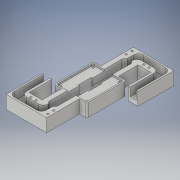
# Autodesk Inventor part: Enclosure_Bottom V6
Saved by Autodesk Inventor 2017 (Build 210142000, 142)
## iProperties
Created: 2017-11-29
Part Number: Enclosure_Bottom V6
Material: Generic
Document SubType Name: Modeling
Designer: Tripl_000
Density: 1 g/cm^3
Appearance: Default
Author: Tripl_000
Autodesk Inventor part; units mm, degrees
ref_plane "YZ Plane" through (0, 0, 0) normal (1, 0, 0) x (0, 1, 0)
ref_plane "XZ Plane" through (0, 0, 0) normal (0, 1, 0) x (-1, 0, 0)
ref_plane "XY Plane" through (0, 0, 0) normal (0, 0, 1) x (1, 0, 0)
sketch "Sketch1" plane through (0, 0, 0) normal (0, 1, 0) x (-1, 0, 0)
  line L0 (-25, 30) -> (25, 30)
  line L1 (25, 30) -> (25, -30)
  line L2 (25, -30) -> (-25, -30)
  line L3 (-25, -30) -> (-25, 30)
  line L4 (-25, 30) -> (25, -30) construction
  line L5 (25, 30) -> (-25, -30) construction
  point P0 (0, 0)
  dimension "d0" = 50
  dimension "d1" = 60
  constraints: 12 end point, 2 midpoint, 2 parallel, 1 horizontal, 1 perpendicular
  measures "d0" distance of L1.end L2.end
  measures "d1" distance of L0.end L1.end
extrude "Extrusion1" add sketch "Sketch1" along normal blind 20
sketch "Sketch2" plane through (-25, 0, 30) normal (0, 0, 1) x (1, 0, 0)
  line L0 (0, 20) -> (50, 20) projected
  line L1 (18.5, 20) -> (31.5, 20)
  line L2 (31.5, 20) -> (31.5, 7)
  line L3 (31.5, 7) -> (18.5, 7)
  line L4 (18.5, 7) -> (18.5, 20)
  line L5 (0, 0) -> (0, 20) projected
  point P0 (25, 0)
  dimension "d4" = 13
  dimension "d5" = 13
  dimension "d6" = 18.5
  constraints: 8 end point, 2 parallel, 1 horizontal, 1 perpendicular, 1 point on line
  measures "d4" distance between parallel lines of L2 L4
  measures "d5" distance between parallel lines of L0 L3
  measures "d6" distance between parallel lines of L4 L5
sketch "Sketch3" plane through (0, 20, 0) normal (0, 1, 0) x (1, 0, 0)
  line L0 (-11.25, 7.5) -> (11.25, 7.5)
  line L1 (11.25, 7.5) -> (11.25, -7.5)
  line L2 (11.25, -7.5) -> (-11.25, -7.5)
  line L3 (-11.25, -7.5) -> (-11.25, 7.5)
  line L4 (-11.25, 7.5) -> (11.25, -7.5) construction
  line L5 (11.25, 7.5) -> (-11.25, -7.5) construction
  point P0 (0, 0)
  dimension "d7" = 22.5
  dimension "d8" = 15
  constraints: 12 end point, 2 midpoint, 2 parallel, 1 horizontal, 1 perpendicular
  measures "d7" distance of L0.start L0.end
  measures "d8" distance between parallel lines of L2 L0
shell "Shell1" thickness 2 removed faces 1 at (-8.3333, 20, -10)
sketch "Sketch4" plane through (-23, 2, 28) normal (0, 1, 0) x (1, 0, 0)
  line L0 (0, 0) -> (0, 56) projected
  line L1 (46, 56) -> (46, 0) projected
  line L2 (0, 56) -> (46, 56)
  line L3 (46, 56) -> (46, 0)
  line L4 (46, 0) -> (0, 0)
  line L5 (0, 0) -> (0, 56)
  point P0 (23, 28)
  constraints: 8 end point, 2 parallel, 1 horizontal, 1 perpendicular
extrude "Extrusion2" add sketch "Sketch4" along normal blind 15.5
extrude "Extrusion3" cut sketch "Sketch3" against normal blind 13
extrude "Extrusion4" cut sketch "Sketch2" against normal through all
sketch "Sketch5" plane through (-23, 17.5, 28) normal (0, 1, 0) x (1, 0, 0)
  circle A0 centre (3, 53) radius 1.5
  line L0 (-27.6389, 28) -> (76.1675, 28)
  line L1 (23, 61.4826) -> (23, -6.2799)
  circle A1 centre (43, 53) radius 1.5
  circle A2 centre (3, 3) radius 1.5
  circle A3 centre (43, 3) radius 1.5
  point P0 (23, 28)
  dimension "d16" = 25
  dimension "d17" = 20
  dimension "d18" = 3
  constraints: 4 centre point, 4 end point, 3 symmetric about line, 1 horizontal, 1 vertical, 3 other
  measures "d16" vertical distance of point (23, 28) A0.centre
  measures "d17" horizontal distance of point (23, 28) A0.centre
  measures "d18" diameter of A0
extrude "Extrusion5" cut sketch "Sketch5" against normal through all
fillet "Fillet1" radius 2 8 edges at (25, 10, 30) (25, 10, -30) (-25, 10, 30) (-25, 10, -30) (-23, 18.75, -28) (23, 18.75, -28) (-23, 18.75, 28) (23, 18.75, 28)
sketch "Sketch6" plane through (-6.5, 7, 30) normal (0, 0, 1) x (1, 0, 0)
  line L0 (20, 13) -> (20, -7)
  line L1 (20, -7) -> (-7, -7)
  line L2 (-7, -7) -> (-7, 13)
  line L3 (-16.5, 13) -> (0, 13) projected
  line L4 (-18.5, 13) -> (-18.5, -7) projected
  line L5 (13, 0) -> (0, 0) projected
  line L6 (0, 13) -> (0, 0)
  line L7 (13, 13) -> (13, 0) projected
  line L8 (0, 0) -> (13, 0)
  line L9 (13, 0) -> (13, 13)
  line L10 (-7, 13) -> (0, 13)
  line L11 (13, 13) -> (20, 13)
  point P0 (6.5, -7)
  dimension "d23" = 11.5
  dimension "d24" = 27
  constraints: 16 end point, 4 perpendicular, 3 parallel, 2 horizontal, 1 collinear
  measures "d23" distance between parallel lines of L4 L2
  measures "d24" distance between parallel lines of L0 L2
extrude "Extrusion6" add sketch "Sketch6" along normal blind 30
sketch "Sketch7" plane through (6.5, 7, -30) normal (0, 0, -1) x (-1, 0, 0)
  line L0 (20, 13) -> (20, -7) projected
  line L1 (20, -7) -> (-7, -7) projected
  line L2 (-7, -7) -> (-7, 13) projected
  line L3 (-7, 13) -> (0, 13) projected
  line L4 (0, 13) -> (0, 0) projected
  line L5 (0, 0) -> (13, 0) projected
  line L6 (13, 0) -> (13, 13) projected
  line L7 (13, 13) -> (20, 13) projected
  point P0 (6.5, -7)
extrude "Extrusion7" add sketch "Sketch7" along normal blind 30
sketch "Sketch8" plane through (6.5, 7, -60) normal (0, 0, -1) x (-1, 0, 0)
  line L0 (-7, -7) -> (-7, 13) projected
  line L1 (20, -7) -> (20, 13) projected
  line L2 (-7, 13) -> (20, 13)
  line L3 (20, 13) -> (20, -7)
  line L4 (20, -7) -> (-7, -7)
  line L5 (-7, -7) -> (-7, 13)
  point P0 (6.5, -7)
  constraints: 8 end point, 2 parallel, 1 horizontal, 1 perpendicular
extrude "Extrusion8" add sketch "Sketch8" along normal blind 20
sketch "Sketch9" plane through (13.5, 0, -30) normal (1, 0, 0) x (0, 0, -1)
  line L0 (50, 0) -> (50, 20) projected
  line L1 (0, 20) -> (50, 20) projected
  line L2 (50, 0) -> (30, 0)
  line L3 (30, 0) -> (30, 20)
  line L4 (30, 20) -> (50, 20)
  line L5 (50, 20) -> (50, 0)
  point P0 (-30, 0)
  dimension "d32" = 20
  constraints: 8 end point, 2 parallel, 1 horizontal, 1 perpendicular, 1 point on line
  measures "d32" distance between parallel lines of L0 L3
extrude "Extrusion9" add sketch "Sketch9" along normal blind 21.5
sketch "Sketch10" plane through (35, 0, -30) normal (1, 0, 0) x (0, 0, -1)
  line L0 (50, 0) -> (50, 20) projected
  line L1 (30, 20) -> (30, 0) projected
  line L2 (50, 0) -> (30, 0)
  line L3 (30, 0) -> (30, 20)
  line L4 (30, 20) -> (50, 20)
  line L5 (50, 20) -> (50, 0)
  point P0 (-30, 0)
  constraints: 8 end point, 2 parallel, 1 horizontal, 1 perpendicular
extrude "Extrusion10" add sketch "Sketch10" along normal blind 13.5
ref_plane "Work Plane1" through (6.5, 7, 0) normal (0, 0, 1) x (1, 0, 0)
mirror "Mirror1" about plane through (6.5, 7, 0) normal (0, 0, 1) of "Extrusion8"
sketch "Sketch11" plane through (-13.5, 0, 30) normal (-1, 0, 0) x (0, 0, 1)
  line L0 (50, 20) -> (50, 0) projected
  line L1 (0, 0) -> (50, 0) projected
  line L2 (50, 20) -> (30, 20)
  line L3 (30, 20) -> (30, 0)
  line L4 (30, 0) -> (50, 0)
  line L5 (50, 0) -> (50, 20)
  point P0 (-30, 0)
  dimension "d38" = 20
  constraints: 8 end point, 2 parallel, 1 horizontal, 1 perpendicular, 1 point on line
  measures "d38" distance of L0.start L2.end
extrude "Extrusion11" add sketch "Sketch11" along normal blind 35
sketch "Sketch12" plane through (13.5, 0, -60) normal (0, 0, 1) x (1, 0, 0)
  line L0 (0, 0) -> (35, 0) projected
  line L1 (0, 20) -> (35, 20) projected
  line L2 (35, 0) -> (20, 0)
  line L3 (20, 0) -> (20, 20)
  line L4 (20, 20) -> (35, 20)
  line L5 (35, 20) -> (35, 0)
  point P0 (-13.5, 0)
  dimension "d41" = 15
  constraints: 8 end point, 2 parallel, 1 horizontal, 1 perpendicular, 1 point on line
  measures "d41" distance between parallel lines of L5 L3
extrude "Extrusion12" add sketch "Sketch12" along normal blind 35
sketch "Sketch13" plane through (-13.5, 0, 60) normal (0, 0, -1) x (-1, 0, 0)
  line L0 (35, 0) -> (35, 20) projected
  line L1 (35, 20) -> (-27, 20) projected
  line L2 (35, 0) -> (20, 0)
  line L3 (20, 0) -> (20, 20)
  line L4 (20, 20) -> (35, 20)
  line L5 (35, 20) -> (35, 0)
  point P0 (-13.5, 0)
  dimension "d44" = 15
  constraints: 8 end point, 2 parallel, 1 horizontal, 1 perpendicular, 1 point on line
  measures "d44" distance between parallel lines of L0 L3
extrude "Extrusion13" add sketch "Sketch13" along normal blind 35
sketch "Sketch14" plane through (6.5, 7, -60) normal (0, 0, 1) x (1, 0, 0)
  line L0 (-9.75, 13) -> (-3.25, 13)
  line L1 (-3.25, 13) -> (-3.25, 0)
  line L2 (-3.25, 0) -> (-9.75, 0)
  line L3 (-9.75, 0) -> (-9.75, 13)
  line L4 (-13, 0) -> (0, 0) projected
  line L5 (0, 0) -> (0, 13) projected
  point P0 (-6.5, -7)
  dimension "d51" = 0
  dimension "d52" = 6.5
  dimension "d53" = 3.25
  dimension "d54" = 13
  constraints: 8 end point, 2 parallel, 1 horizontal, 1 perpendicular
  measures "d51" distance between parallel lines of L4 L2
  measures "d52" distance between parallel lines of L1 L3
  measures "d53" distance between parallel lines of L5 L1
  measures "d54" distance of L2.end L0.start
extrude "Extrusion14" cut sketch "Sketch14" against normal blind 17.5
mirror "Mirror2" about plane through (6.5, 7, 0) normal (0, 0, 1) of "Extrusion14"
sketch "Sketch15" plane through (3.25, 7, -60) normal (-1, 0, 0) x (0, 0, 1)
  line L0 (-17.5, 13) -> (-17.5, 0) projected
  line L1 (-17.5, 0) -> (-8.5, 0)
  line L2 (-8.5, 0) -> (-8.5, 13)
  line L3 (-8.5, 13) -> (-17.5, 13)
  line L4 (-17.5, 13) -> (-17.5, 0)
  point P0 (60, -7)
  dimension "d61" = 13
  dimension "d62" = 9
  constraints: 8 end point, 2 parallel, 1 horizontal, 1 perpendicular
  measures "d61" distance of L1.end L2.end
  measures "d62" distance of L2.end L3.end
extrude "Extrusion15" cut sketch "Sketch15" against normal blind 43
sketch "Sketch16" plane through (3.25, 7, -68.5) normal (0, 0, -1) x (-1, 0, 0)
  line L0 (-43, 13) -> (-33.5, 13)
  line L1 (-33.5, 13) -> (-33.5, 0)
  line L2 (-33.5, 0) -> (-43, 0)
  line L3 (-43, 0) -> (-43, 13)
  line L4 (0, 0) -> (-43, 0) projected
  line L5 (-43, 13) -> (-43, 0) projected
  point P0 (3.25, -7)
  dimension "d73" = 9.5
  dimension "d74" = 0
  dimension "d75" = 0
  dimension "d76" = 13
  constraints: 8 end point, 2 parallel, 1 horizontal, 1 perpendicular
  measures "d73" distance of L0.start L0.end
  measures "d74" distance between parallel lines of L4 L2
  measures "d75" distance between parallel lines of L5 L3
  measures "d76" distance of L0.end L1.end
extrude "Extrusion16" cut sketch "Sketch16" against normal through all
sketch "Sketch17" plane through (-3.25, 7, 60) normal (1, 0, 0) x (0, 0, -1)
  line L0 (-17.5, 0) -> (-8, 0)
  line L1 (-8, 0) -> (-8, 13)
  line L2 (-8, 13) -> (-17.5, 13)
  line L3 (-17.5, 13) -> (-17.5, 0)
  point P0 (60, -7)
  dimension "d83" = 13
  dimension "d84" = 9.5
  constraints: 8 end point, 2 parallel, 1 horizontal, 1 perpendicular
  measures "d83" distance of L0.end L1.end
  measures "d84" distance of L1.end L2.end
extrude "Extrusion17" cut sketch "Sketch17" against normal blind 43
sketch "Sketch18" plane through (-3.25, 7, 68) normal (0, 0, 1) x (1, 0, 0)
  line L0 (0, 0) -> (-43, 0) projected
  line L1 (-43, 0) -> (-33.5, 0)
  line L2 (-33.5, 0) -> (-33.5, 13)
  line L3 (-33.5, 13) -> (-43, 13)
  line L4 (-43, 13) -> (-43, 0)
  point P0 (3.25, -7)
  dimension "d91" = 13
  dimension "d92" = 9.5
  constraints: 8 end point, 2 parallel, 1 horizontal, 1 perpendicular
  measures "d91" distance of L1.end L2.end
  measures "d92" distance of L2.end L3.end
extrude "Extrusion18" cut sketch "Sketch18" against normal through all
fillet "Fillet2" radius 7.5 8 edges at (-46.25, 13.5, 77.5) (-36.75, 13.5, 68) (3.25, 13.5, 77.5) (-3.25, 13.5, 68) (-3.25, 13.5, -77.5) (3.25, 13.5, -68.5) (46.25, 13.5, -77.5) (36.75, 13.5, -68.5)
fillet "Fillet3" radius 5 4 edges at (-6.5, 13.5, 60) (6.5, 13.5, 60) (-6.5, 13.5, -60) (6.5, 13.5, -60)
sketch "Sketch19" plane through (0, 20, 0) normal (0, 1, 0) x (1, 0, 0)
  circle A0 centre (17.5, 65) radius 1.5
  circle A1 centre (25.5, 65) radius 1.5
  circle A2 centre (-9.5, 74) radius 1.5
  circle A3 centre (-9.5, 65) radius 1.5
  circle A4 centre (9.5, -74) radius 1.5
  circle A5 centre (9.5, -65) radius 1.5
  circle A6 centre (-25.5, -65) radius 1.5
  circle A7 centre (-17.5, -65) radius 1.5
  line L0 (13.5, 60) -> (33.5, 60) projected
  line L1 (13.5, 30) -> (13.5, 60) projected
  line L2 (-13.5, -30) -> (-13.5, -60) projected
  line L3 (-13.5, -60) -> (-33.5, -60) projected
  line L4 (-13.5, 30) -> (-13.5, 80) projected
  line L5 (13.5, -30) -> (13.5, -80) projected
  line L6 (-48.5, -80) -> (13.5, -80) projected
  line L7 (-13.5, 80) -> (48.5, 80) projected
  point P0 (0, 0)
  dimension "d97" = 5
  dimension "d98" = 5
  dimension "d99" = 4
  dimension "d100" = 12
  dimension "d101" = 3
  dimension "d102" = 3
  dimension "d103" = 4
  dimension "d104" = 12
  dimension "d105" = 5
  dimension "d106" = 5
  dimension "d107" = 3
  dimension "d108" = 3
  dimension "d109" = 4
  dimension "d110" = 4
  dimension "d111" = 4
  dimension "d112" = 4
  dimension "d113" = 6
  dimension "d114" = 15
  dimension "d115" = 6
  dimension "d116" = 15
  dimension "d117" = 3
  dimension "d118" = 3
  dimension "d119" = 3
  dimension "d120" = 3
  constraints: 8 centre point
  measures "d97" distance from line of A0.centre L0
  measures "d98" distance from line of L0 A1.centre
  measures "d99" distance from line of L1 A0.centre
  measures "d100" distance from line of L1 A1.centre
  measures "d101" diameter of A0
  measures "d102" diameter of A1
  measures "d103" distance from line of L2 A7.centre
  measures "d104" distance from line of L2 A6.centre
  measures "d105" distance from line of A6.centre L3
  measures "d106" distance from line of A7.centre L3
  measures "d107" diameter of A6
  measures "d108" diameter of A7
  measures "d109" distance from line of A3.centre L4
  measures "d110" distance from line of A2.centre L4
  measures "d111" distance from line of A5.centre L5
  measures "d112" distance from line of A4.centre L5
  measures "d113" distance from line of A4.centre L6
  measures "d114" distance from line of A5.centre L6
  measures "d115" distance from line of A2.centre L7
  measures "d116" distance from line of A3.centre L7
  measures "d117" diameter of A2
  measures "d118" diameter of A3
  measures "d119" diameter of A5
  measures "d120" diameter of A4
extrude "Extrusion19" cut sketch "Sketch19" against normal through all
sketch "Sketch20" plane through (-23, 17.5, 28) normal (0, 1, 0) x (1, 0, 0)
  line L0 (16.5, 20.5) -> (11.75, 20.5) projected
  line L1 (11.75, 35.5) -> (16.5, 35.5) projected
  line L2 (11.75, 20.5) -> (14.75, 20.5)
  line L3 (14.75, 20.5) -> (14.75, 35.5)
  line L4 (14.75, 35.5) -> (11.75, 35.5)
  line L5 (11.75, 35.5) -> (11.75, 20.5)
  line L6 (23, -121.2558) -> (23, 233.7966)
  point P0 (23, 28)
  dimension "d123" = 3
  constraints: 10 end point, 2 parallel, 1 horizontal, 1 perpendicular, 1 point on line, 1 vertical
  measures "d123" distance between parallel lines of L3 L5
extrude "Extrusion20" add sketch "Sketch20" against normal up to surface (10.5 mm away)
ref_plane "Work Plane2" through (0, 7, 7.5) normal (1, 0, 0) x (0, 0, -1)
mirror "Mirror3" about plane through (0, 7, 7.5) normal (1, 0, 0) of "Extrusion20"
sketch "Sketch21" plane through (-23, 17.5, 28) normal (0, 1, 0) x (1, 0, 0)
  line L0 (16.5, 0) -> (16.5, 20.5) projected
  line L1 (16.5, 18) -> (14.75, 18)
  line L2 (14.75, 18) -> (14.75, 38)
  line L3 (14.75, 38) -> (16.5, 38)
  line L4 (16.5, 38) -> (16.5, 18)
  line L5 (16.5, 20.5) -> (14.75, 20.5) projected
  line L6 (14.75, 35.5) -> (16.5, 35.5) projected
  line L7 (23, -99.3518) -> (23, 163.4818)
  line L8 (29.5, 18) -> (31.25, 18)
  line L9 (31.25, 18) -> (31.25, 38)
  line L10 (31.25, 38) -> (29.5, 38)
  line L11 (29.5, 38) -> (29.5, 18)
  point P0 (23, 28)
  dimension "d127" = 1.75
  dimension "d128" = 2.5
  dimension "d129" = 2.5
  constraints: 18 end point, 4 symmetric about line, 2 parallel, 1 horizontal, 1 perpendicular, 1 point on line, 1 vertical
  measures "d127" distance of L2.end L3.end
  measures "d128" distance between parallel lines of L5 L1
  measures "d129" distance between parallel lines of L3 L6
extrude "Extrusion21" cut sketch "Sketch21" against normal blind 16.5
sketch "Sketch22" plane through (0, 7, 0) normal (0, 1, 0) x (1, 0, 0)
  line L0 (-8.25, 10) -> (-6.5, 10) projected
  line L1 (6.5, -10) -> (-6.5, -10)
  line L2 (-6.5, -10) -> (-6.5, 10)
  line L3 (-6.5, 10) -> (6.5, 10)
  line L4 (6.5, 10) -> (6.5, -10)
  line L5 (6.5, -10) -> (-6.5, 10) construction
  line L6 (-6.5, -10) -> (6.5, 10) construction
  point P0 (0, 0)
  constraints: 12 end point, 2 midpoint, 2 parallel, 1 horizontal, 1 perpendicular
extrude "Extrusion22" cut sketch "Sketch22" against normal up to surface (6 mm away)
body "Solid1"
